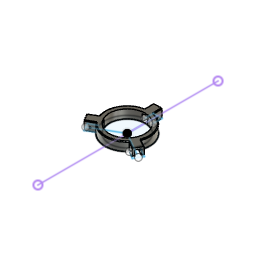
Tripod1 v1 (Autodesk Fusion 360 design; units mm, degrees)
Autodesk Fusion 360 part; units mm, degrees
sketch "Sketch1" plane through (0, 0, 0) normal (0, 0, 1) x (1, 0, 0)
  circle A0 centre (0, 0) radius 41
  line L0 (-10, 50.01) -> (-10, 70.01)
  line L1 (-10, 70.01) -> (10, 70.01)
  line L2 (10, 70.01) -> (10, 50.01)
  line L3 (0, 0) -> (0, 70.01)
  line L4 (0, 0) -> (60.6304, -35.005)
  line L5 (0, 0) -> (-60.6304, -35.005)
  line L6 (48.3099, -16.3447) -> (65.6304, -26.3447)
  line L7 (65.6304, -26.3447) -> (55.6304, -43.6653)
  line L8 (55.6304, -43.6653) -> (38.3099, -33.6653)
  arc A1 (48.3099, -16.3447) -> (10, 50.01) centre (0, 0) ccw
  line L9 (-38.3099, -33.6653) -> (-55.6304, -43.6653)
  line L10 (-55.6304, -43.6653) -> (-65.6304, -26.3447)
  line L11 (-65.6304, -26.3447) -> (-48.3099, -16.3447)
  arc A2 (-10, 50.01) -> (-48.3099, -16.3447) centre (0, 0) ccw
  arc A3 (-38.3099, -33.6653) -> (38.3099, -33.6653) centre (0, 0) ccw
  line L12 (0, -205.75) -> (0, 209.25)
  dimension "d1" = 82
  dimension "d2" = 102
  dimension "d3" = 20
  dimension "d4" = 20
  dimension "d5" = 70.01
  dimension "d6" = 120
  dimension "d7" = 70.01
  dimension "d8" = 70.01
  dimension "d9" = 120
  dimension "d10" = 20
  dimension "d11" = 20
  dimension "d12" = 20
  dimension "d13" = 20
  dimension "d14" = 20
  dimension "d15" = 20
  constraint coincident A0.centre L3.start
  constraint coincident L0.start A2.start
  constraint vertical L0
  constraint perpendicular L0 L1
  constraint coincident L2.end A1.end
  constraint perpendicular L1 L2
  constraint midpoint L1 L3.end
  constraint coincident L6.start A2
  constraint symmetric L4 L6.start L8.end
  constraint coincident L6.start A1.start
  constraint parallel L4 L6
  constraint perpendicular L6 L7
  constraint coincident L8.end A3.end
  constraint concentric A1 A2
  constraint coincident L9.start A2
  constraint symmetric L5 L9.start L11.end
  constraint coincident L9.start A3.start
  constraint parallel L5 L9
  constraint perpendicular L9 L10
  constraint coincident L11.end A2.end
  constraint concentric A2 A3
  measures "d1" diameter of A0
  measures "d2" diameter of A2
  measures "d3" distance of L0.start L2.end
  measures "d4" distance of L0.start L0.end
  measures "d5" distance of A0.centre L4.end
  measures "d6" angle of L3 L4
  measures "d7" distance of A0.centre L3.end
  measures "d8" distance of A0.centre L5.end
  measures "d9" angle of L3 L5
  measures "d10" distance of L6.start L8.end
  measures "d11" distance of L6.start L6.end
  measures "d12" distance of L6.end L7.end
  measures "d13" distance of L9.start L11.end
  measures "d14" distance of L9.start L9.end
  measures "d15" distance of L9.end L10.end
extrude "Extrude1" add sketch "Sketch1" along normal blind 20 contours A0 L1 L2 L3 L4 L6 L7 A1 L12 | A0 L0 L1 L3 L5 L10 L11 A2 L12 | A0 L4 L7 L8 A3 L12 | A0 L5 L9 L10 A3 L12
sketch "Sketch2" plane through (0, 0, 0) normal (0, 0, -1) x (1, 0, 0)
  circle A0 centre (0, 0) radius 41
  line L0 (-38.3099, 33.6653) -> (-55.6304, 43.6653)
  line L1 (-55.6304, 43.6653) -> (-65.6304, 26.3447)
  line L2 (-65.6304, 26.3447) -> (-48.3099, 16.3447)
  arc A1 (-48.3099, 16.3447) -> (-10, -50.01) centre (0, 0) ccw
  line L3 (-10, -50.01) -> (-10, -70.01)
  line L4 (-10, -70.01) -> (10, -70.01)
  line L5 (10, -70.01) -> (10, -50.01)
  arc A2 (10, -50.01) -> (48.3099, 16.3447) centre (0, 0) ccw
  line L6 (48.3099, 16.3447) -> (65.6304, 26.3447)
  line L7 (65.6304, 26.3447) -> (55.6304, 43.6653)
  line L8 (55.6304, 43.6653) -> (38.3099, 33.6653)
  arc A3 (38.3099, 33.6653) -> (-38.3099, 33.6653) centre (0, 0) ccw
  line L9 (-6, -40.5586) -> (-6, -70.01)
  line L10 (-6, -70.01) -> (6, -70.01)
  line L11 (6, -70.01) -> (6, -40.5586)
  line L12 (0, 0) -> (0, -70.01)
  line L13 (-10, -70.01) -> (10, -70.01)
  circle A4 centre (0, 0) radius 41
  line L14 (-38.1248, 15.0831) -> (-32.1248, 25.4755)
  line L15 (-32.1248, 25.4755) -> (-57.6304, 40.2012)
  line L16 (-57.6304, 40.2012) -> (-63.6304, 29.8088)
  line L17 (-63.6304, 29.8088) -> (-38.1248, 15.0831)
  line L18 (0, 0) -> (-60.6304, 35.005)
  line L19 (38.1248, 15.0831) -> (32.1248, 25.4755)
  line L20 (32.1248, 25.4755) -> (57.6304, 40.2012)
  line L21 (57.6304, 40.2012) -> (63.6304, 29.8088)
  line L22 (63.6304, 29.8088) -> (38.1248, 15.0831)
  line L23 (0, 0) -> (60.6304, 35.005)
  dimension "d18" = 12
  dimension "d19" = 70.01
  dimension "d20" = 70.01
  dimension "d21" = 70.01
  dimension "d22" = 12
  dimension "d23" = 70.01
  dimension "d24" = 12
  constraint parallel L9 L11
  constraint coincident A0 L9.start
  constraint coincident A0 L11.end
  constraint perpendicular L14 L15
  constraint parallel L14 L16
  constraint parallel L15 L17
  constraint coincident A4 L14.end
  constraint coincident A0 L14.start
  constraint symmetric L15 L17 L18
  constraint perpendicular L19 L20
  constraint parallel L19 L21
  constraint parallel L20 L22
  constraint coincident A4 L19.end
  constraint coincident A4 L19.start
  constraint symmetric L20 L22 L23
  constraint perpendicular L9 L10
  measures "d18" distance of L9 L11
  measures "d19" distance of L13 A0.centre
  measures "d20" distance of L10 A0.centre
  measures "d21" distance of A0.centre L16
  measures "d22" distance of L15.end L16.end
  measures "d23" distance of L21 A0.centre
  measures "d24" distance of L20 L22
extrude "Extrude2" cut sketch "Sketch2" against normal blind 16 contours A0 L7 A4 L21 L22 L23 | A0 L4 L10 L11 L12 L13 A4 | A0 L7 A4 L20 L21 L23 | A0 L4 L9 L10 L12 L13 A4 | A0 L1 A4 L15 L16 L18 | A0 L1 A4 L16 L17 L18
sketch "Sketch3" plane through (10, 0, 0) normal (1, 0, 0) x (0, 1, 0)
  line L0 (50.01, 0) -> (70.01, 0)
  line L1 (70.01, 0) -> (70.01, 20)
  line L2 (70.01, 20) -> (50.01, 20)
  line L3 (50.01, 20) -> (50.01, 0)
  line L4 (40.5586, 16) -> (70.01, 16)
  circle A0 centre (60.01, 8) radius 1.6
  point P0 (60.01, 8)
  dimension "d27" = 8
  dimension "d28" = 10
  dimension "d29" = 3.2
  constraint coincident P0 A0.centre
  measures "d27" distance of P0 L4
  measures "d28" distance of L3 P0
  measures "d29" diameter of A0
extrude "Extrude3" cut sketch "Sketch3" along normal through all and the other way through all contours A0
sketch "Sketch4" plane through (5, 8.6603, 0) normal (0.5, 0.866025, 0) x (-0.866025, 0.5, 0)
  line L0 (-70.01, 0) -> (-50.01, 0)
  line L1 (-50.01, 0) -> (-50.01, 20)
  line L2 (-50.01, 20) -> (-70.01, 20)
  line L3 (-70.01, 20) -> (-70.01, 0)
  line L4 (-70.01, 16) -> (-40.5586, 16)
  circle A0 centre (-60.01, 8) radius 1.6
  point P0 (-60.01, 8)
  dimension "d32" = 8
  dimension "d33" = 10
  dimension "d34" = 3.2
  constraint coincident P0 A0.centre
  measures "d32" distance of P0 L4
  measures "d33" distance of L3 P0
  measures "d34" diameter of A0
extrude "Extrude4" cut sketch "Sketch4" along normal through all and the other way through all contours A0
sketch "Sketch5" plane through (5, -8.6603, 0) normal (0.5, -0.866025, 0) x (0.866025, 0.5, 0)
  line L0 (-70.01, 0) -> (-50.01, 0)
  line L1 (-50.01, 0) -> (-50.01, 20)
  line L2 (-50.01, 20) -> (-70.01, 20)
  line L3 (-70.01, 20) -> (-70.01, 0)
  line L4 (-70.01, 16) -> (-40.5586, 16)
  circle A0 centre (-60.01, 8) radius 1.6
  point P0 (-60.01, 8)
  dimension "d37" = 10
  dimension "d38" = 8
  dimension "d39" = 3.2
  constraint coincident P0 A0.centre
  measures "d37" distance of L3 P0
  measures "d38" distance of P0 L4
  measures "d39" diameter of A0
extrude "Extrude5" cut sketch "Sketch5" along normal through all and the other way through all contours A0
fillet "Fillet1" radius 1.5 9 edges at (0, -51, 20) (46.9702, -38.6653, 20) (56.9702, -21.3447, 20) (44.1673, 25.5, 20) (10, 60.01, 20) (-10, 60.01, 20) (-44.1673, 25.5, 20) (-56.9702, -21.3447, 20) (-46.9702, -38.6653, 20)
fillet "Fillet2" radius 5 6 edges at (-64.6304, -28.0768, 0) (-56.6304, -41.9332, 0) (-8, 70.01, 0) (8, 70.01, 0) (56.6304, -41.9332, 0) (64.6304, -28.0768, 0)
equation "d5 = d7"
equation "d8 = d7"
equation "d20 = d19"
equation "d21 = d19"
equation "d23 = d19"
